Autodesk Fusion 360 part; units mm, degrees
note: some values were not read from the file. Set by a fixed rule: which sketch regions a step uses.
(part 3 of 8)
  spline S676 degree 3 poles (21.5017, -36.3646) (20.0626, -38.8974) (15.4509, -40.8816) (15.3621, -42.4125) knots 0 0 0 0 1 1 1 1
  spline S677 degree 3 poles (50.353, -26.1302) (50.6772, -26.1304) (51.0587, -26.408) (51.0577, -26.8365) knots 0 0 0 0 1 1 1 1
  spline S678 degree 3 poles (51.0577, -26.8365) (51.0567, -27.2899) (50.7639, -27.6151) (50.3584, -27.6166) knots 0 0 0 0 1 1 1 1
  spline S679 degree 3 poles (50.3584, -27.6166) (49.9248, -27.6184) (49.616, -27.2356) (49.6086, -26.8743) knots 0 0 0 0 1 1 1 1
  spline S680 degree 3 poles (49.6086, -26.8743) (49.5995, -26.4269) (49.9201, -26.13) (50.353, -26.1302) knots 0 0 0 0 1 1 1 1
  spline S681 degree 3 poles (51.5406, -53.5633) (51.8647, -53.5635) (52.2462, -53.8411) (52.2453, -54.2696) knots 0 0 0 0 1 1 1 1
  spline S682 degree 3 poles (52.2453, -54.2696) (52.2443, -54.723) (51.9515, -55.0482) (51.546, -55.0497) knots 0 0 0 0 1 1 1 1
  spline S683 degree 3 poles (51.546, -55.0497) (51.1123, -55.0515) (50.8035, -54.6687) (50.7962, -54.3074) knots 0 0 0 0 1 1 1 1
  spline S684 degree 3 poles (50.7962, -54.3074) (50.787, -53.86) (51.1077, -53.5631) (51.5406, -53.5633) knots 0 0 0 0 1 1 1 1
  spline S685 degree 3 poles (72.4312, -14.4997) (76.2469, -14.5855) (80.5372, -17.3952) (80.5274, -22.9562) knots 0 0 0 0 1 1 1 1
  spline S686 degree 3 poles (80.5274, -22.9562) (80.5194, -27.4888) (76.2962, -31.0017) (72.6195, -30.8225) knots 0 0 0 0 1 1 1 1
  spline S687 degree 3 poles (72.6195, -30.8225) (67.4693, -30.5715) (64.6367, -26.4712) (64.4292, -22.1695) knots 0 0 0 0 1 1 1 1
  spline S688 degree 3 poles (64.4292, -22.1695) (64.2167, -17.7617) (68.8119, -14.4186) (72.4312, -14.4997) knots 0 0 0 0 1 1 1 1
  spline S689 degree 3 poles (74.5023, -39.3772) (78.318, -39.4629) (82.6083, -42.2726) (82.5985, -47.8336) knots 0 0 0 0 1 1 1 1
  spline S690 degree 3 poles (82.5985, -47.8336) (82.5905, -52.3663) (78.3672, -55.8792) (74.6906, -55.7) knots 0 0 0 0 1 1 1 1
  spline S691 degree 3 poles (74.6906, -55.7) (69.5404, -55.449) (66.7077, -51.3486) (66.5003, -47.0469) knots 0 0 0 0 1 1 1 1
  spline S692 degree 3 poles (66.5003, -47.0469) (66.2878, -42.6392) (70.883, -39.2961) (74.5023, -39.3772) knots 0 0 0 0 1 1 1 1
  spline S693 degree 3 poles (73.2785, -58.2074) (82.3005, -57.5327) (89.9582, -48.2547) (90.1203, -35.5662) knots 0 0 0 0 1 1 1 1
  spline S694 degree 2 poles (90.1203, -35.5662) (87.4866, -35.4301) (84.6007, -35.3111) knots 0 0 0 1 1 1
  line L146 (84.6007, -35.3111) -> (84.471, -32.0483)
  spline S695 degree 2 poles (84.471, -32.0483) (87.0415, -31.8252) (89.6592, -31.806) knots 0 0 0 1 1 1
  spline S696 degree 3 poles (89.6592, -31.806) (89.4171, -23.0769) (80.9156, -11.9731) (70.8766, -11.9613) knots 0 0 0 0 1 1 1 1
  spline S697 degree 3 poles (70.8766, -11.9613) (65.914, -11.9571) (60.8467, -16.8048) (60.6556, -22.2308) knots 0 0 0 0 1 1 1 1
  spline S698 degree 3 poles (60.6556, -22.2308) (60.4942, -26.8139) (64.4737, -30.3857) (65.4815, -34.4267) knots 0 0 0 0 1 1 1 1
  spline S699 degree 2 poles (65.4815, -34.4267) (66.1184, -34.46) (67.0382, -34.426) knots 0 0 0 1 1 1
  line L147 (67.0382, -34.426) -> (67.0737, -37.0293)
  spline S700 degree 2 poles (67.0737, -37.0293) (65.9901, -37.0984) (65.537, -37.0984) knots 0 0 0 1 1 1
  spline S701 degree 3 poles (65.537, -37.0984) (65.3316, -41.8108) (62.9469, -42.7703) (63.0893, -47.5705) knots 0 0 0 0 1 1 1 1
  spline S702 degree 3 poles (63.0893, -47.5705) (63.3075, -54.9251) (68.8259, -58.3029) (73.2785, -58.2074) knots 0 0 0 0 1 1 1 1
  spline S703 degree 3 poles (75.2555, -32.5471) (76.3242, -32.5305) (77.1113, -32.4934) (78.4498, -32.4976) knots 0 0 0 0 1 1 1 1
  spline S704 degree 3 poles (78.4498, -32.4976) (79.3002, -32.4997) (79.9929, -33.259) (80.0372, -34.5532) knots 0 0 0 0 1 1 1 1
  spline S705 degree 3 poles (80.0372, -34.5532) (80.0711, -35.5384) (79.5067, -36.6633) (78.5769, -36.7117) knots 0 0 0 0 1 1 1 1
  spline S706 degree 3 poles (78.5769, -36.7117) (77.3189, -36.7771) (76.4003, -36.7367) (74.9094, -36.745) knots 0 0 0 0 1 1 1 1
  spline S707 degree 3 poles (74.9094, -36.745) (73.8775, -36.7492) (73.3711, -35.5379) (73.3735, -34.5911) knots 0 0 0 0 1 1 1 1
  spline S708 degree 3 poles (73.3735, -34.5911) (73.3763, -33.5178) (73.9925, -32.5674) (75.2555, -32.549) knots 0 0 0 0 1 1 1 1
  line L148 (75.2555, -32.549) -> (75.2555, -32.5471)
  spline S709 degree 3 poles (23.3685, -73.0015) (22.2201, -71.8744) (21.4826, -70.2942) (21.3371, -68.6485) knots 0 0 0 0 1 1 1 1
  spline S710 degree 3 poles (21.3371, -68.6485) (21.2174, -67.2961) (21.5085, -65.8738) (22.2993, -64.8005) knots 0 0 0 0 1 1 1 1
  spline S711 degree 3 poles (22.2993, -64.8005) (22.6948, -64.2639) (23.2101, -63.822) (23.7995, -63.5458) knots 0 0 0 0 1 1 1 1
  spline S712 degree 3 poles (23.7995, -63.5458) (24.3889, -63.2696) (25.0523, -63.1624) (25.6902, -63.2644) knots 0 0 0 0 1 1 1 1
  spline S713 degree 3 poles (25.6902, -63.2644) (25.9412, -63.3046) (26.1875, -63.3765) (26.4223, -63.4781) knots 0 0 0 0 1 1 1 1
  line L149 (26.4223, -63.4781) -> (26.3432, -66.5101)
  spline S714 degree 3 poles (26.3432, -66.5101) (26.3414, -66.5806) (26.3399, -66.6516) (26.3518, -66.721) knots 0 0 0 0 1 1 1 1
  spline S715 degree 3 poles (26.3518, -66.721) (26.3636, -66.7904) (26.3893, -66.8584) (26.4339, -66.9111) knots 0 0 0 0 1 1 1 1
  spline S716 degree 3 poles (26.4339, -66.9111) (26.4838, -66.97) (26.5544, -67.0063) (26.6274, -67.0245) knots 0 0 0 0 1 1 1 1
  spline S717 degree 3 poles (26.6274, -67.0245) (26.7003, -67.0427) (26.7761, -67.044) (26.851, -67.0447) knots 0 0 0 0 1 1 1 1
  line L150 (26.851, -67.0447) -> (30.6238, -67.0829)
  spline S718 degree 3 poles (30.6238, -67.0829) (30.7378, -67.084) (30.852, -67.0875) (30.9657, -67.078) knots 0 0 0 0 1 1 1 1
  spline S719 degree 3 poles (30.9657, -67.078) (31.0793, -67.0685) (31.1951, -67.0436) (31.2905, -66.9778) knots 0 0 0 0 1 1 1 1
  spline S720 degree 3 poles (31.2905, -66.9778) (31.3594, -66.9303) (31.4152, -66.8619) (31.4495, -66.7831) knots 0 0 0 0 1 1 1 1
  spline S721 degree 3 poles (31.4495, -66.7831) (31.4838, -66.7042) (31.4964, -66.615) (31.4855, -66.5291) knots 0 0 0 0 1 1 1 1
  line L151 (31.4855, -66.5291) -> (31.5307, -64.1427)
  spline S722 degree 3 poles (31.5307, -64.1427) (31.5118, -64.0654) (31.5145, -63.9824) (31.5385, -63.9067) knots 0 0 0 0 1 1 1 1
  spline S723 degree 3 poles (31.5385, -63.9067) (31.5625, -63.8309) (31.6077, -63.7628) (31.6669, -63.7129) knots 0 0 0 0 1 1 1 1
  spline S724 degree 3 poles (31.6669, -63.7129) (31.7303, -63.6596) (31.8081, -63.6279) (31.8876, -63.6109) knots 0 0 0 0 1 1 1 1
  spline S725 degree 3 poles (31.8876, -63.6109) (31.9671, -63.5939) (32.0486, -63.5911) (32.1296, -63.5886) knots 0 0 0 0 1 1 1 1
  line L152 (32.1296, -63.5886) -> (36.4643, -63.4554)
  spline S726 degree 3 poles (36.4643, -63.4554) (36.4791, -62.6007) (36.898, -61.7642) (37.5596, -61.2684) knots 0 0 0 0 1 1 1 1
  spline S727 degree 3 poles (37.5596, -61.2684) (37.8482, -61.052) (38.1798, -60.9005) (38.5261, -60.8212) knots 0 0 0 0 1 1 1 1
  spline S728 degree 3 poles (38.5261, -60.8212) (38.8723, -60.7419) (39.2297, -60.7387) (39.584, -60.7443) knots 0 0 0 0 1 1 1 1
  line L153 (39.584, -60.7443) -> (51.3262, -60.9286)
  spline S729 degree 3 poles (51.3262, -60.9286) (51.8918, -60.9406) (52.451, -61.1692) (52.8762, -61.562) knots 0 0 0 0 1 1 1 1
  spline S730 degree 3 poles (52.8762, -61.562) (53.2339, -61.8924) (53.4915, -62.3265) (53.7043, -62.7746) knots 0 0 0 0 1 1 1 1
  spline S731 degree 3 poles (53.7043, -62.7746) (53.8166, -63.011) (53.9182, -63.2535) (54.0434, -63.4826) knots 0 0 0 0 1 1 1 1
  spline S732 degree 3 poles (54.0434, -63.4826) (54.1686, -63.7117) (54.3195, -63.9292) (54.5148, -64.0953) knots 0 0 0 0 1 1 1 1
  spline S733 degree 3 poles (54.5148, -64.0953) (54.8537, -64.3832) (55.2965, -64.4935) (55.727, -64.5627) knots 0 0 0 0 1 1 1 1
  spline S734 degree 3 poles (55.727, -64.5627) (56.3986, -64.6707) (57.0794, -64.6956) (57.7585, -64.7155) knots 0 0 0 0 1 1 1 1
  line L154 (57.7585, -64.7155) -> (115.2201, -66.3956)
  spline S735 degree 3 poles (115.2201, -66.3956) (115.6074, -66.4069) (115.9977, -66.4549) (116.381, -66.3956) knots 0 0 0 0 1 1 1 1
  spline S736 degree 3 poles (116.381, -66.3956) (116.6412, -66.3553) (116.8939, -66.2531) (117.1065, -66.0901) knots 0 0 0 0 1 1 1 1
  spline S737 degree 3 poles (117.1065, -66.0901) (117.5006, -65.7881) (117.7284, -65.3094) (117.9771, -64.8682) knots 0 0 0 0 1 1 1 1
  spline S738 degree 3 poles (117.9771, -64.8682) (118.2594, -64.3676) (118.5967, -63.8834) (119.0603, -63.5661) knots 0 0 0 0 1 1 1 1
  spline S739 degree 3 poles (119.0603, -63.5661) (119.4759, -63.2816) (119.982, -63.1465) (120.4761, -63.1881) knots 0 0 0 0 1 1 1 1
  line L155 (120.4761, -63.1881) -> (132.583, -63.5028)
  spline S740 degree 3 poles (132.583, -63.5028) (133.2403, -63.4478) (133.9156, -63.7151) (134.3755, -64.2125) knots 0 0 0 0 1 1 1 1
  spline S741 degree 3 poles (134.3755, -64.2125) (134.8733, -64.7509) (135.1048, -65.5483) (134.9778, -66.2876) knots 0 0 0 0 1 1 1 1
  line L156 (134.9778, -66.2876) -> (139.3853, -66.5036)
  spline S742 degree 3 poles (139.3853, -66.5036) (139.5114, -66.5097) (139.6383, -66.5162) (139.7611, -66.5467) knots 0 0 0 0 1 1 1 1
  spline S743 degree 3 poles (139.7611, -66.5467) (139.8839, -66.5773) (140.0037, -66.6337) (140.0932, -66.7273) knots 0 0 0 0 1 1 1 1
  spline S744 degree 3 poles (140.0932, -66.7273) (140.1909, -66.8294) (140.2466, -66.9694) (140.2731, -67.1117) knots 0 0 0 0 1 1 1 1
  spline S745 degree 3 poles (140.2731, -67.1117) (140.2995, -67.2539) (140.299, -67.4) (140.2984, -67.545) knots 0 0 0 0 1 1 1 1
  line L157 (140.2984, -67.545) -> (140.2899, -69.7019)
  spline S746 degree 3 poles (140.2899, -69.7019) (140.2895, -69.8149) (140.2888, -69.9287) (140.3062, -70.0402) knots 0 0 0 0 1 1 1 1
  spline S747 degree 3 poles (140.3062, -70.0402) (140.3237, -70.1518) (140.3608, -70.2625) (140.4299, -70.3491) knots 0 0 0 0 1 1 1 1
  spline S748 degree 3 poles (140.4299, -70.3491) (140.4775, -70.4086) (140.5395, -70.4552) (140.6085, -70.4833) knots 0 0 0 0 1 1 1 1
  spline S749 degree 3 poles (140.6085, -70.4833) (140.6774, -70.5113) (140.7531, -70.5207) (140.8264, -70.5103) knots 0 0 0 0 1 1 1 1
  line L158 (140.8264, -70.5103) -> (144.5244, -70.5643)
  spline S750 degree 3 poles (144.5244, -70.5643) (144.685, -70.5887) (144.8549, -70.5347) (144.9758, -70.4208) knots 0 0 0 0 1 1 1 1
  spline S751 degree 3 poles (144.9758, -70.4208) (145.114, -70.2906) (145.1837, -70.0845) (145.1546, -69.8917) knots 0 0 0 0 1 1 1 1
  line L159 (145.1546, -69.8917) -> (145.2484, -67.1238)
  spline S752 degree 3 poles (145.2484, -67.1238) (145.4352, -66.9982) (145.6371, -66.8973) (145.8476, -66.8242) knots 0 0 0 0 1 1 1 1
  spline S753 degree 3 poles (145.8476, -66.8242) (146.4322, -66.6212) (147.0785, -66.639) (147.6628, -66.8426) knots 0 0 0 0 1 1 1 1
  spline S754 degree 3 poles (147.6628, -66.8426) (148.2471, -67.0463) (148.769, -67.4308) (149.1755, -67.9173) knots 0 0 0 0 1 1 1 1
  spline S755 degree 3 poles (149.1755, -67.9173) (149.9885, -68.8903) (150.3196, -70.2311) (150.3052, -71.5268) knots 0 0 0 0 1 1 1 1
  spline S756 degree 3 poles (150.3052, -71.5268) (150.2851, -73.328) (149.627, -75.1136) (148.4877, -76.4578) knots 0 0 0 0 1 1 1 1
  line L160 (148.4877, -76.4578) -> (134.4681, -76.4409)
  spline S757 degree 3 poles (134.4681, -76.4409) (134.3422, -76.9072) (134.0363, -77.3167) (133.6355, -77.5556) knots 0 0 0 0 1 1 1 1
  spline S758 degree 3 poles (133.6355, -77.5556) (133.3442, -77.7292) (133.0111, -77.813) (132.6779, -77.848) knots 0 0 0 0 1 1 1 1
  spline S759 degree 3 poles (132.6779, -77.848) (132.3448, -77.8829) (132.009, -77.8712) (131.6744, -77.8603) knots 0 0 0 0 1 1 1 1
  line L161 (131.6744, -77.8603) -> (116.3387, -77.3573)
  spline S760 degree 3 poles (116.3387, -77.3573) (116.1319, -77.3505) (115.9238, -77.3446) (115.7192, -77.3771) knots 0 0 0 0 1 1 1 1
  spline S761 degree 3 poles (115.7192, -77.3771) (115.5146, -77.4095) (115.3125, -77.4818) (115.1471, -77.6126) knots 0 0 0 0 1 1 1 1
  spline S762 degree 3 poles (115.1471, -77.6126) (115.0025, -77.727) (114.8892, -77.8848) (114.8241, -78.0624) knots 0 0 0 0 1 1 1 1
  spline S763 degree 3 poles (114.8241, -78.0624) (114.7589, -78.24) (114.7422, -78.437) (114.7763, -78.624) knots 0 0 0 0 1 1 1 1
  line L162 (114.7763, -78.624) -> (114.7162, -87.671)
  spline S764 degree 3 poles (114.7162, -87.671) (114.6628, -88.1799) (114.8565, -88.7106) (115.2197, -89.0511) knots 0 0 0 0 1 1 1 1
  spline S765 degree 3 poles (115.2197, -89.0511) (115.4965, -89.3106) (115.8654, -89.4587) (116.2362, -89.4591) knots 0 0 0 0 1 1 1 1
  line L163 (116.2362, -89.4591) -> (132.4279, -90.0963)
  spline S766 degree 3 poles (132.4279, -90.0963) (132.8986, -90.0815) (133.3726, -90.2466) (133.7419, -90.5541) knots 0 0 0 0 1 1 1 1
  spline S767 degree 3 poles (133.7419, -90.5541) (134.1545, -90.8976) (134.4311, -91.4166) (134.4945, -91.9662) knots 0 0 0 0 1 1 1 1
  line L164 (134.4945, -91.9662) -> (148.1256, -92.4599)
  spline S768 degree 3 poles (148.1256, -92.4599) (148.8324, -93.2896) (149.3295, -94.3154) (149.5527, -95.4047) knots 0 0 0 0 1 1 1 1
  spline S769 degree 3 poles (149.5527, -95.4047) (149.7758, -96.4941) (149.7244, -97.6444) (149.4052, -98.7069) knots 0 0 0 0 1 1 1 1
  spline S770 degree 3 poles (149.4052, -98.7069) (149.0854, -99.7712) (148.4747, -100.7686) (147.5774, -101.3635) knots 0 0 0 0 1 1 1 1
  spline S771 degree 3 poles (147.5774, -101.3635) (146.721, -101.9313) (145.6312, -102.0927) (144.6592, -101.7955) knots 0 0 0 0 1 1 1 1
  line L165 (144.6592, -101.7955) -> (144.5317, -98.7315)
  spline S772 degree 3 poles (144.5317, -98.7315) (144.494, -98.5283) (144.3864, -98.3402) (144.2334, -98.21) knots 0 0 0 0 1 1 1 1
  spline S773 degree 3 poles (144.2334, -98.21) (144.0917, -98.0894) (143.9121, -98.0189) (143.73, -98.0125) knots 0 0 0 0 1 1 1 1
  line L166 (143.73, -98.0125) -> (139.8707, -98.0758)
  spline S774 degree 3 poles (139.8707, -98.0758) (139.7838, -98.054) (139.6903, -98.0623) (139.6081, -98.099) knots 0 0 0 0 1 1 1 1
  spline S775 degree 3 poles (139.6081, -98.099) (139.5259, -98.1358) (139.4553, -98.2008) (139.4098, -98.2817) knots 0 0 0 0 1 1 1 1
  spline S776 degree 3 poles (139.4098, -98.2817) (139.3572, -98.3752) (139.3389, -98.4893) (139.3592, -98.5957) knots 0 0 0 0 1 1 1 1
  line L167 (139.3592, -98.5957) -> (139.3379, -101.0866)
  spline S777 degree 3 poles (139.3379, -101.0866) (139.337, -101.196) (139.3371, -101.306) (139.3207, -101.414) knots 0 0 0 0 1 1 1 1
  spline S778 degree 3 poles (139.3207, -101.414) (139.3042, -101.522) (139.2689, -101.6303) (139.199, -101.7111) knots 0 0 0 0 1 1 1 1
  spline S779 degree 3 poles (139.199, -101.7111) (139.1442, -101.7743) (139.0692, -101.8179) (138.9892, -101.833) knots 0 0 0 0 1 1 1 1
  spline S780 degree 3 poles (138.9892, -101.833) (138.9092, -101.8482) (138.8245, -101.8348) (138.7523, -101.7955) knots 0 0 0 0 1 1 1 1
  line L168 (138.7523, -101.7955) -> (134.2379, -101.7601)
  spline S781 degree 3 poles (134.2379, -101.7601) (134.2725, -102.4664) (133.9962, -103.1829) (133.5036, -103.6639) knots 0 0 0 0 1 1 1 1
  spline S782 degree 3 poles (133.5036, -103.6639) (132.998, -104.1575) (132.2742, -104.3924) (131.5923, -104.2841) knots 0 0 0 0 1 1 1 1
  line L169 (131.5923, -104.2841) -> (119.2583, -103.9786)
  spline S783 degree 3 poles (119.2583, -103.9786) (118.7444, -103.8806) (118.2487, -103.6772) (117.8073, -103.3832) knots 0 0 0 0 1 1 1 1
  spline S784 degree 3 poles (117.8073, -103.3832) (116.7983, -102.7111) (116.0967, -101.5504) (115.9458, -100.3036) knots 0 0 0 0 1 1 1 1
  line L170 (115.9458, -100.3036) -> (56.2679, -98.6327)
  spline S785 degree 3 poles (56.2679, -98.6327) (55.8319, -98.6205) (55.3941, -98.5951) (54.9602, -98.6429) knots 0 0 0 0 1 1 1 1
  spline S786 degree 3 poles (54.9602, -98.6429) (54.6434, -98.6777) (54.328, -98.7575) (54.0452, -98.9117) knots 0 0 0 0 1 1 1 1
  spline S787 degree 3 poles (54.0452, -98.9117) (53.7463, -99.0747) (53.4855, -99.3242) (53.3294, -99.6382) knots 0 0 0 0 1 1 1 1
  spline S788 degree 3 poles (53.3294, -99.6382) (53.1481, -100.0025) (53.1141, -100.4327) (52.9316, -100.7963) knots 0 0 0 0 1 1 1 1
  spline S789 degree 3 poles (52.9316, -100.7963) (52.8073, -101.0437) (52.6153, -101.2529) (52.3847, -101.3923) knots 0 0 0 0 1 1 1 1
  spline S790 degree 3 poles (52.3847, -101.3923) (52.1541, -101.5316) (51.8857, -101.6006) (51.62, -101.5888) knots 0 0 0 0 1 1 1 1
  line L171 (51.62, -101.5888) -> (38.2822, -101.4082)
  spline S791 degree 3 poles (38.2822, -101.4082) (38.1033, -101.4058) (37.9235, -101.3983) (37.7488, -101.358) knots 0 0 0 0 1 1 1 1
  spline S792 degree 3 poles (37.7488, -101.358) (37.5741, -101.3177) (37.4064, -101.2475) (37.2488, -101.1583) knots 0 0 0 0 1 1 1 1
  spline S793 degree 3 poles (37.2488, -101.1583) (36.8107, -100.9104) (36.4463, -100.5206) (36.2178, -100.0555) knots 0 0 0 0 1 1 1 1
  spline S794 degree 3 poles (36.2178, -100.0555) (35.9894, -99.5904) (35.8979, -99.052) (35.959, -98.5324) knots 0 0 0 0 1 1 1 1
  line L172 (35.959, -98.5324) -> (31.6131, -98.6049)
  spline S795 degree 3 poles (31.6131, -98.6049) (31.5119, -98.6066) (31.4103, -98.6079) (31.3101, -98.5929) knots 0 0 0 0 1 1 1 1
  spline S796 degree 3 poles (31.3101, -98.5929) (31.2099, -98.5779) (31.1108, -98.5463) (31.0254, -98.4892) knots 0 0 0 0 1 1 1 1
  spline S797 degree 3 poles (31.0254, -98.4892) (30.9406, -98.4325) (30.8709, -98.3512) (30.826, -98.2566) knots 0 0 0 0 1 1 1 1
  spline S798 degree 3 poles (30.826, -98.2566) (30.7811, -98.1621) (30.7611, -98.0546) (30.7689, -97.9492) knots 0 0 0 0 1 1 1 1
  line L173 (30.7689, -97.9492) -> (30.5725, -95.1552)
  spline S799 degree 3 poles (30.5725, -95.1552) (30.5791, -94.9521) (30.5069, -94.7475) (30.3761, -94.5982) knots 0 0 0 0 1 1 1 1
  spline S800 degree 3 poles (30.3761, -94.5982) (30.2413, -94.4444) (30.0457, -94.3515) (29.847, -94.3467) knots 0 0 0 0 1 1 1 1
  line L174 (29.847, -94.3467) -> (26.5432, -94.3467)
  spline S801 degree 3 poles (26.5432, -94.3467) (26.3535, -94.3319) (26.1591, -94.414) (26.0317, -94.5627) knots 0 0 0 0 1 1 1 1
  spline S802 degree 3 poles (26.0317, -94.5627) (25.9082, -94.707) (25.8501, -94.9108) (25.8778, -95.1027) knots 0 0 0 0 1 1 1 1
  line L175 (25.8778, -95.1027) -> (25.9042, -98.2099)
  spline S803 degree 3 poles (25.9042, -98.2099) (25.7162, -98.2716) (25.5234, -98.3171) (25.3283, -98.3457) knots 0 0 0 0 1 1 1 1
  spline S804 degree 3 poles (25.3283, -98.3457) (24.1437, -98.5197) (22.9086, -98.0401) (22.0479, -97.1659) knots 0 0 0 0 1 1 1 1
  spline S805 degree 3 poles (22.0479, -97.1659) (21.1872, -96.2916) (20.694, -95.0535) (20.6085, -93.7977) knots 0 0 0 0 1 1 1 1
  spline S806 degree 3 poles (20.6085, -93.7977) (20.5409, -92.8051) (20.7186, -91.795) (21.1194, -90.8936) knots 0 0 0 0 1 1 1 1
  spline S807 degree 3 poles (21.1194, -90.8936) (21.5202, -89.9923) (22.1432, -89.2016) (22.9106, -88.6204) knots 0 0 0 0 1 1 1 1
  line L176 (22.9106, -88.6204) -> (36.0543, -88.6414)
  spline S808 degree 3 poles (36.0543, -88.6414) (36.2423, -88.3197) (36.4933, -88.039) (36.7871, -87.8221) knots 0 0 0 0 1 1 1 1
  spline S809 degree 3 poles (36.7871, -87.8221) (37.3131, -87.4338) (37.9769, -87.2578) (38.6149, -87.3376) knots 0 0 0 0 1 1 1 1
  line L177 (38.6149, -87.3376) -> (54.2246, -87.6077)
  spline S810 degree 3 poles (54.2246, -87.6077) (54.4295, -87.6112) (54.6346, -87.618) (54.8393, -87.6072) knots 0 0 0 0 1 1 1 1
  spline S811 degree 3 poles (54.8393, -87.6072) (55.044, -87.5964) (55.2513, -87.5652) (55.4368, -87.4734) knots 0 0 0 0 1 1 1 1
  spline S812 degree 3 poles (55.4368, -87.4734) (55.6027, -87.3914) (55.7466, -87.2608) (55.8483, -87.1003) knots 0 0 0 0 1 1 1 1
  spline S813 degree 3 poles (55.8483, -87.1003) (55.9499, -86.9398) (56.009, -86.7497) (56.0172, -86.557) knots 0 0 0 0 1 1 1 1
  line L178 (56.0172, -86.557) -> (56.1022, -76.9699)
  spline S814 degree 3 poles (56.1022, -76.9699) (56.1428, -76.6491) (56.0582, -76.3127) (55.8721, -76.0551) knots 0 0 0 0 1 1 1 1
  spline S815 degree 3 poles (55.8721, -76.0551) (55.7532, -75.8904) (55.5945, -75.7579) (55.4151, -75.6734) knots 0 0 0 0 1 1 1 1
  spline S816 degree 3 poles (55.4151, -75.6734) (55.2358, -75.589) (55.0361, -75.5527) (54.8403, -75.5691) knots 0 0 0 0 1 1 1 1
  line L179 (54.8403, -75.5691) -> (39.2114, -75.1109)
  spline S817 degree 3 poles (39.2114, -75.1109) (38.6875, -75.1125) (38.1643, -74.941) (37.7339, -74.6265) knots 0 0 0 0 1 1 1 1
  spline S818 degree 3 poles (37.7339, -74.6265) (37.2427, -74.2675) (36.8765, -73.7231) (36.7182, -73.1161) knots 0 0 0 0 1 1 1 1
  line L180 (36.7182, -73.1161) -> (23.3685, -73.0015)
  spline S819 degree 3 poles (61.6296, -85.4421) (62.5295, -85.7248) (63.5344, -85.6159) (64.3607, -85.1461) knots 0 0 0 0 1 1 1 1
  spline S820 degree 3 poles (64.3607, -85.1461) (65.1869, -84.6762) (65.8243, -83.8512) (66.0929, -82.904) knots 0 0 0 0 1 1 1 1
  spline S821 degree 3 poles (66.0929, -82.904) (66.3616, -81.9568) (66.2581, -80.899) (65.8117, -80.0293) knots 0 0 0 0 1 1 1 1
  spline S822 degree 3 poles (65.8117, -80.0293) (65.3653, -79.1596) (64.5816, -78.4887) (63.6817, -78.2059) knots 0 0 0 0 1 1 1 1
  spline S823 degree 3 poles (63.6817, -78.2059) (62.7818, -77.9232) (61.7769, -78.0321) (60.9507, -78.5019) knots 0 0 0 0 1 1 1 1
  spline S824 degree 3 poles (60.9507, -78.5019) (60.1244, -78.9718) (59.487, -79.7968) (59.2184, -80.744) knots 0 0 0 0 1 1 1 1
  spline S825 degree 3 poles (59.2184, -80.744) (58.9498, -81.6912) (59.0533, -82.749) (59.4996, -83.6187) knots 0 0 0 0 1 1 1 1
  spline S826 degree 3 poles (59.4996, -83.6187) (59.946, -84.4884) (60.7297, -85.1593) (61.6296, -85.4421) knots 0 0 0 0 1 1 1 1
  spline S827 degree 3 poles (107.0839, -86.9677) (107.9838, -87.2504) (108.9887, -87.1415) (109.815, -86.6716) knots 0 0 0 0 1 1 1 1
  spline S828 degree 3 poles (109.815, -86.6716) (110.6412, -86.2018) (111.2786, -85.3768) (111.5472, -84.4296) knots 0 0 0 0 1 1 1 1
  spline S829 degree 3 poles (111.5472, -84.4296) (111.8159, -83.4824) (111.7124, -82.4246) (111.266, -81.5549) knots 0 0 0 0 1 1 1 1
  spline S830 degree 3 poles (111.266, -81.5549) (110.8196, -80.6852) (110.0359, -80.0142) (109.136, -79.7315) knots 0 0 0 0 1 1 1 1
  spline S831 degree 3 poles (109.136, -79.7315) (108.2362, -79.4487) (107.2312, -79.5577) (106.405, -80.0275) knots 0 0 0 0 1 1 1 1
  spline S832 degree 3 poles (106.405, -80.0275) (105.5787, -80.4973) (104.9413, -81.3223) (104.6727, -82.2695) knots 0 0 0 0 1 1 1 1
  spline S833 degree 3 poles (104.6727, -82.2695) (104.4041, -83.2168) (104.5076, -84.2745) (104.9539, -85.1443) knots 0 0 0 0 1 1 1 1
  spline S834 degree 3 poles (104.9539, -85.1443) (105.4003, -86.014) (106.1841, -86.6849) (107.0839, -86.9677) knots 0 0 0 0 1 1 1 1
  spline S835 degree 3 poles (70.4371, -72.9822) (70.1477, -72.9883) (69.8625, -73.1192) (69.6613, -73.3381) knots 0 0 0 0 1 1 1 1
  spline S836 degree 3 poles (69.6613, -73.3381) (69.46, -73.557) (69.3451, -73.8613) (69.3488, -74.1659) knots 0 0 0 0 1 1 1 1
  spline S837 degree 3 poles (69.3488, -74.1659) (69.3517, -74.4139) (69.4321, -74.6603) (69.5745, -74.8579) knots 0 0 0 0 1 1 1 1
  spline S838 degree 3 poles (69.5745, -74.8579) (69.717, -75.0556) (69.9207, -75.2034) (70.1468, -75.2732) knots 0 0 0 0 1 1 1 1
  line L181 (70.1468, -75.2732) -> (100.9091, -75.9224)
  spline S839 degree 3 poles (100.9091, -75.9224) (101.1096, -75.8838) (101.2987, -75.7822) (101.4459, -75.634) knots 0 0 0 0 1 1 1 1
  spline S840 degree 3 poles (101.4459, -75.634) (101.5931, -75.4857) (101.698, -75.2914) (101.7435, -75.0823) knots 0 0 0 0 1 1 1 1
  spline S841 degree 3 poles (101.7435, -75.0823) (101.8202, -74.73) (101.7196, -74.3405) (101.4841, -74.0775) knots 0 0 0 0 1 1 1 1
  spline S842 degree 3 poles (101.4841, -74.0775) (101.2485, -73.8145) (100.885, -73.686) (100.5464, -73.7459) knots 0 0 0 0 1 1 1 1
  line L182 (100.5464, -73.7459) -> (99.6395, -73.7077)
  line L183 (99.6395, -73.7077) -> (99.6757, -74.1277)
  line L184 (99.6757, -74.1277) -> (97.6806, -74.1277)
  line L185 (97.6806, -74.1277) -> (97.6806, -73.6695)
  line L186 (97.6806, -73.6695) -> (96.0118, -73.6313)
  line L187 (96.0118, -73.6313) -> (96.0118, -74.0895)
  line L188 (96.0118, -74.0895) -> (93.8715, -74.0895)
  line L189 (93.8715, -74.0895) -> (93.8353, -73.5549)
  line L190 (93.8353, -73.5549) -> (92.2391, -73.5549)
  line L191 (92.2391, -73.5549) -> (92.2391, -74.0513)
  line L192 (92.2391, -74.0513) -> (90.1351, -73.9749)
  line L193 (90.1351, -73.9749) -> (90.1714, -73.4785)
  line L194 (90.1714, -73.4785) -> (88.6115, -73.4022)
  line L195 (88.6115, -73.4022) -> (88.6115, -73.8604)
  line L196 (88.6115, -73.8604) -> (86.5437, -73.784)
  line L197 (86.5437, -73.784) -> (86.5437, -73.364)
  line L198 (86.5437, -73.364) -> (84.8025, -73.364)
  line L199 (84.8025, -73.364) -> (84.8387, -73.7459)
  line L200 (84.8387, -73.7459) -> (82.6984, -73.6313)
  line L201 (82.6984, -73.6313) -> (82.6984, -73.1731)
  line L202 (82.6984, -73.1731) -> (81.0297, -73.1349)
  line L203 (81.0297, -73.1349) -> (81.0297, -73.6313)
  line L204 (81.0297, -73.6313) -> (78.9983, -73.5931)
  line L205 (78.9983, -73.5931) -> (79.0345, -73.1349)
  line L206 (79.0345, -73.1349) -> (77.1119, -73.1349)
  line L207 (77.1119, -73.1349) -> (77.1482, -73.5549)
  line L208 (77.1482, -73.5549) -> (75.1892, -73.4786)
  line L209 (75.1892, -73.4786) -> (75.1892, -73.0203)
  line L210 (75.1892, -73.0203) -> (73.3754, -72.9822)
  line L211 (73.3754, -72.9822) -> (73.3754, -73.4404)
  line L212 (73.3754, -73.4404) -> (71.4528, -73.4022)
  line L213 (71.4528, -73.4022) -> (71.4891, -72.9822)
  line L214 (71.4891, -72.9822) -> (70.4371, -72.9822)
  spline S843 degree 3 poles (70.2066, -88.9065) (69.9173, -88.9126) (69.6321, -89.0435) (69.4308, -89.2624) knots 0 0 0 0 1 1 1 1
  spline S844 degree 3 poles (69.4308, -89.2624) (69.2296, -89.4813) (69.1147, -89.7856) (69.1183, -90.0902) knots 0 0 0 0 1 1 1 1
  spline S845 degree 3 poles (69.1183, -90.0902) (69.1213, -90.3383) (69.2016, -90.5846) (69.3441, -90.7823) knots 0 0 0 0 1 1 1 1
  spline S846 degree 3 poles (69.3441, -90.7823) (69.4865, -90.9799) (69.6902, -91.1277) (69.9164, -91.1976) knots 0 0 0 0 1 1 1 1
  line L215 (69.9164, -91.1976) -> (100.6787, -91.8467)
  spline S847 degree 3 poles (100.6787, -91.8467) (100.8791, -91.8081) (101.0682, -91.7065) (101.2154, -91.5583) knots 0 0 0 0 1 1 1 1
  spline S848 degree 3 poles (101.2154, -91.5583) (101.3627, -91.41) (101.4675, -91.2157) (101.513, -91.0066) knots 0 0 0 0 1 1 1 1
  spline S849 degree 3 poles (101.513, -91.0066) (101.5897, -90.6544) (101.4892, -90.2648) (101.2536, -90.0018) knots 0 0 0 0 1 1 1 1
  spline S850 degree 3 poles (101.2536, -90.0018) (101.0181, -89.7389) (100.6545, -89.6103) (100.3159, -89.6702) knots 0 0 0 0 1 1 1 1
  line L216 (100.3159, -89.6702) -> (99.409, -89.632)
  line L217 (99.409, -89.632) -> (99.4453, -90.052)
  line L218 (99.4453, -90.052) -> (97.4501, -90.052)
  line L219 (97.4501, -90.052) -> (97.4501, -89.5938)
  line L220 (97.4501, -89.5938) -> (95.7814, -89.5556)
  line L221 (95.7814, -89.5556) -> (95.7814, -90.0138)
  line L222 (95.7814, -90.0138) -> (93.6411, -90.0138)
  line L223 (93.6411, -90.0138) -> (93.6048, -89.4792)
  line L224 (93.6048, -89.4792) -> (92.0087, -89.4792)
  line L225 (92.0087, -89.4792) -> (92.0087, -89.9756)
  line L226 (92.0087, -89.9756) -> (89.9046, -89.8993)
  line L227 (89.9046, -89.8993) -> (89.9409, -89.4029)
  line L228 (89.9409, -89.4029) -> (88.381, -89.3265)
  line L229 (88.381, -89.3265) -> (88.381, -89.7847)
  line L230 (88.381, -89.7847) -> (86.3133, -89.7084)
  line L231 (86.3133, -89.7084) -> (86.3133, -89.2883)
  line L232 (86.3133, -89.2883) -> (84.572, -89.2883)
  line L233 (84.572, -89.2883) -> (84.6083, -89.6702)
  line L234 (84.6083, -89.6702) -> (82.468, -89.5556)
  line L235 (82.468, -89.5556) -> (82.468, -89.0974)
  line L236 (82.468, -89.0974) -> (80.7993, -89.0592)
  line L237 (80.7993, -89.0592) -> (80.7993, -89.5556)
  line L238 (80.7993, -89.5556) -> (78.7678, -89.5174)
  line L239 (78.7678, -89.5174) -> (78.8041, -89.0592)
  line L240 (78.8041, -89.0592) -> (76.8814, -89.0592)
  line L241 (76.8814, -89.0592) -> (76.9177, -89.4792)
  line L242 (76.9177, -89.4792) -> (74.9588, -89.4029)
  line L243 (74.9588, -89.4029) -> (74.9588, -88.9447)
  line L244 (74.9588, -88.9447) -> (73.145, -88.9065)
  line L245 (73.145, -88.9065) -> (73.145, -89.3647)
  line L246 (73.145, -89.3647) -> (71.2223, -89.3265)
  line L247 (71.2223, -89.3265) -> (71.2586, -88.9065)
  line L248 (71.2586, -88.9065) -> (70.2066, -88.9065)
  spline S851 degree 3 poles (40.0515, -65.8778) (39.9072, -65.8671) (39.7599, -65.9107) (39.6421, -65.9989) knots 0 0 0 0 1 1 1 1
  spline S852 degree 3 poles (39.6421, -65.9989) (39.5107, -66.0973) (39.4176, -66.2509) (39.3882, -66.4178) knots 0 0 0 0 1 1 1 1
  line L249 (39.3882, -66.4178) -> (39.3644, -69.1877)
  spline S853 degree 3 poles (39.3644, -69.1877) (39.3568, -69.3937) (39.43, -69.6017) (39.5633, -69.7528) knots 0 0 0 0 1 1 1 1
  spline S854 degree 3 poles (39.5633, -69.7528) (39.7182, -69.9283) (39.9524, -70.0225) (40.179, -70.0004) knots 0 0 0 0 1 1 1 1
  line L250 (40.179, -70.0004) -> (49.3108, -69.9688)
  spline S855 degree 3 poles (49.3108, -69.9688) (49.7498, -69.8504) (50.1478, -69.5705) (50.4197, -69.1889) knots 0 0 0 0 1 1 1 1
  spline S856 degree 3 poles (50.4197, -69.1889) (50.6917, -68.8074) (50.8357, -68.3268) (50.8209, -67.8501) knots 0 0 0 0 1 1 1 1
  spline S857 degree 3 poles (50.8209, -67.8501) (50.8061, -67.3735) (50.6327, -66.9039) (50.3379, -66.5419) knots 0 0 0 0 1 1 1 1
  spline S858 degree 3 poles (50.3379, -66.5419) (50.043, -66.1798) (49.6286, -65.9278) (49.1833, -65.8396) knots 0 0 0 0 1 1 1 1
  line L251 (49.1833, -65.8396) -> (40.0515, -65.8778)
  spline S859 degree 3 poles (39.4762, -92.3793) (39.332, -92.3686) (39.1847, -92.4122) (39.0669, -92.5004) knots 0 0 0 0 1 1 1 1
  spline S860 degree 3 poles (39.0669, -92.5004) (38.9354, -92.5989) (38.8424, -92.7524) (38.8129, -92.9193) knots 0 0 0 0 1 1 1 1
  line L252 (38.8129, -92.9193) -> (38.7891, -95.6892)
  spline S861 degree 3 poles (38.7891, -95.6892) (38.7816, -95.8952) (38.8548, -96.1032) (38.9881, -96.2543) knots 0 0 0 0 1 1 1 1
  spline S862 degree 3 poles (38.9881, -96.2543) (39.1429, -96.4298) (39.3771, -96.524) (39.6037, -96.5019) knots 0 0 0 0 1 1 1 1
  line L253 (39.6037, -96.5019) -> (48.7355, -96.4703)
  spline S863 degree 3 poles (48.7355, -96.4703) (49.1745, -96.3519) (49.5725, -96.072) (49.8445, -95.6904) knots 0 0 0 0 1 1 1 1
  spline S864 degree 3 poles (49.8445, -95.6904) (50.1164, -95.3089) (50.2604, -94.8284) (50.2456, -94.3516) knots 0 0 0 0 1 1 1 1
  spline S865 degree 3 poles (50.2456, -94.3516) (50.2309, -93.875) (50.0575, -93.4054) (49.7626, -93.0434) knots 0 0 0 0 1 1 1 1
  spline S866 degree 3 poles (49.7626, -93.0434) (49.4677, -92.6813) (49.0533, -92.4293) (48.608, -92.3411) knots 0 0 0 0 1 1 1 1
  line L254 (48.608, -92.3411) -> (39.4762, -92.3793)
  spline S867 degree 3 poles (120.9407, -94.9113) (120.7967, -94.8988) (120.6488, -94.9405) (120.53, -95.0272) knots 0 0 0 0 1 1 1 1
  spline S868 degree 3 poles (120.53, -95.0272) (120.3975, -95.124) (120.3027, -95.2763) (120.2713, -95.4429) knots 0 0 0 0 1 1 1 1
  line L255 (120.2713, -95.4429) -> (120.2157, -98.2123)
  spline S869 degree 3 poles (120.2157, -98.2123) (120.2061, -98.4182) (120.2766, -98.6271) (120.4082, -98.7799) knots 0 0 0 0 1 1 1 1
  spline S870 degree 3 poles (120.4082, -98.7799) (120.561, -98.9573) (120.7941, -99.0545) (121.0209, -99.0353) knots 0 0 0 0 1 1 1 1
  line L256 (121.0209, -99.0353) -> (130.1525, -99.1196)
  spline S871 degree 3 poles (130.1525, -99.1196) (130.5927, -99.0068) (130.994, -98.732) (131.2703, -98.3539) knots 0 0 0 0 1 1 1 1
  spline S872 degree 3 poles (131.2703, -98.3539) (131.5465, -97.9758) (131.696, -97.4971) (131.6867, -97.0203) knots 0 0 0 0 1 1 1 1
  spline S873 degree 3 poles (131.6867, -97.0203) (131.6772, -96.5435) (131.5094, -96.0717) (131.2187, -95.706) knots 0 0 0 0 1 1 1 1
  spline S874 degree 3 poles (131.2187, -95.706) (130.928, -95.3402) (130.5165, -95.0829) (130.0723, -94.9891) knots 0 0 0 0 1 1 1 1
  line L257 (130.0723, -94.9891) -> (120.9407, -94.9113)
  spline S875 degree 3 poles (121.5841, -68.169) (121.4392, -68.1599) (121.2917, -68.2048) (121.1739, -68.2942) knots 0 0 0 0 1 1 1 1
  spline S876 degree 3 poles (121.1739, -68.2942) (121.0371, -68.3981) (120.9423, -68.5614) (120.917, -68.737) knots 0 0 0 0 1 1 1 1
  line L258 (120.917, -68.737) -> (120.8736, -71.6787)
  spline S877 degree 3 poles (120.8736, -71.6787) (120.8582, -71.8959) (120.9304, -72.1184) (121.0686, -72.2805) knots 0 0 0 0 1 1 1 1
  spline S878 degree 3 poles (121.0686, -72.2805) (121.2216, -72.4599) (121.4537, -72.5613) (121.6824, -72.5487) knots 0 0 0 0 1 1 1 1
  line L259 (121.6824, -72.5487) -> (130.8142, -72.5912)
  spline S879 degree 3 poles (130.8142, -72.5912) (131.2614, -72.4454) (131.6609, -72.1424) (131.9338, -71.742) knots 0 0 0 0 1 1 1 1
  spline S880 degree 3 poles (131.9338, -71.742) (132.2067, -71.3416) (132.3514, -70.8462) (132.3393, -70.3536) knots 0 0 0 0 1 1 1 1
  spline S881 degree 3 poles (132.3393, -70.3536) (132.3272, -69.8627) (132.1596, -69.3775) (131.8692, -68.9932) knots 0 0 0 0 1 1 1 1
  spline S882 degree 3 poles (131.8692, -68.9932) (131.5789, -68.6088) (131.1676, -68.3276) (130.716, -68.2046) knots 0 0 0 0 1 1 1 1
  line L260 (130.716, -68.2046) -> (121.5841, -68.169)
  spline S883 degree 3 poles (50.9385, -73.4216) (50.7451, -73.3668) (50.5295, -73.3948) (50.3608, -73.5083) knots 0 0 0 0 1 1 1 1
  spline S884 degree 3 poles (50.3608, -73.5083) (50.2764, -73.5651) (50.2043, -73.6422) (50.1531, -73.7327) knots 0 0 0 0 1 1 1 1
  spline S885 degree 3 poles (50.1531, -73.7327) (50.1018, -73.8233) (50.0718, -73.9272) (50.0679, -74.0325) knots 0 0 0 0 1 1 1 1
  spline S886 degree 3 poles (50.0679, -74.0325) (50.0641, -74.1357) (50.0855, -74.2395) (50.128, -74.3325) knots 0 0 0 0 1 1 1 1
  spline S887 degree 3 poles (50.128, -74.3325) (50.1706, -74.4255) (50.2342, -74.5075) (50.3113, -74.5713) knots 0 0 0 0 1 1 1 1
  spline S888 degree 3 poles (50.3113, -74.5713) (50.4655, -74.6989) (50.6719, -74.7499) (50.866, -74.7198) knots 0 0 0 0 1 1 1 1
  spline S889 degree 3 poles (50.866, -74.7198) (51.0123, -74.6972) (51.1533, -74.6293) (51.2598, -74.5212) knots 0 0 0 0 1 1 1 1
  spline S890 degree 3 poles (51.2598, -74.5212) (51.3663, -74.4131) (51.4366, -74.2643) (51.4464, -74.1089) knots 0 0 0 0 1 1 1 1
  spline S891 degree 3 poles (51.4464, -74.1089) (51.4562, -73.952) (51.404, -73.7933) (51.3102, -73.6709) knots 0 0 0 0 1 1 1 1
  spline S892 degree 3 poles (51.3102, -73.6709) (51.2164, -73.5486) (51.0828, -73.4624) (50.9385, -73.4216) knots 0 0 0 0 1 1 1 1
  spline S893 degree 3 poles (50.6842, -88.2085) (50.4908, -88.1537) (50.2752, -88.1817) (50.1065, -88.2952) knots 0 0 0 0 1 1 1 1
  spline S894 degree 3 poles (50.1065, -88.2952) (50.0221, -88.352) (49.95, -88.4291) (49.8987, -88.5196) knots 0 0 0 0 1 1 1 1
  spline S895 degree 3 poles (49.8987, -88.5196) (49.8475, -88.6102) (49.8174, -88.7141) (49.8136, -88.8194) knots 0 0 0 0 1 1 1 1
  spline S896 degree 3 poles (49.8136, -88.8194) (49.8097, -88.9226) (49.8311, -89.0264) (49.8737, -89.1194) knots 0 0 0 0 1 1 1 1
  spline S897 degree 3 poles (49.8737, -89.1194) (49.9163, -89.2124) (49.9799, -89.2944) (50.057, -89.3582) knots 0 0 0 0 1 1 1 1
  spline S898 degree 3 poles (50.057, -89.3582) (50.2112, -89.4858) (50.4176, -89.5368) (50.6116, -89.5068) knots 0 0 0 0 1 1 1 1
  spline S899 degree 3 poles (50.6116, -89.5068) (50.758, -89.4841) (50.899, -89.4162) (51.0055, -89.3081) knots 0 0 0 0 1 1 1 1
  spline S900 degree 3 poles (51.0055, -89.3081) (51.112, -89.2) (51.1823, -89.0512) (51.1921, -88.8958) knots 0 0 0 0 1 1 1 1
  spline S901 degree 3 poles (51.1921, -88.8958) (51.2019, -88.7389) (51.1497, -88.5802) (51.0559, -88.4578) knots 0 0 0 0 1 1 1 1
  spline S902 degree 3 poles (51.0559, -88.4578) (50.962, -88.3355) (50.8284, -88.2493) (50.6842, -88.2085) knots 0 0 0 0 1 1 1 1
  spline S903 degree 3 poles (120.117, -75.6839) (119.9237, -75.6291) (119.7081, -75.6572) (119.5393, -75.7706) knots 0 0 0 0 1 1 1 1
  spline S904 degree 3 poles (119.5393, -75.7706) (119.455, -75.8274) (119.3828, -75.9045) (119.3316, -75.9951) knots 0 0 0 0 1 1 1 1
  spline S905 degree 3 poles (119.3316, -75.9951) (119.2804, -76.0856) (119.2503, -76.1895) (119.2464, -76.2948) knots 0 0 0 0 1 1 1 1
  spline S906 degree 3 poles (119.2464, -76.2948) (119.2422, -76.398) (119.264, -76.5018) (119.3066, -76.5948) knots 0 0 0 0 1 1 1 1
  spline S907 degree 3 poles (119.3066, -76.5948) (119.3492, -76.6878) (119.4128, -76.7698) (119.4899, -76.8336) knots 0 0 0 0 1 1 1 1
  spline S908 degree 3 poles (119.4899, -76.8336) (119.644, -76.9612) (119.8505, -77.0122) (120.0445, -76.9822) knots 0 0 0 0 1 1 1 1
  spline S909 degree 3 poles (120.0445, -76.9822) (120.1909, -76.9595) (120.3319, -76.8916) (120.4384, -76.7835) knots 0 0 0 0 1 1 1 1
  spline S910 degree 3 poles (120.4384, -76.7835) (120.5449, -76.6754) (120.6152, -76.5266) (120.6249, -76.3712) knots 0 0 0 0 1 1 1 1
  spline S911 degree 3 poles (120.6249, -76.3712) (120.6345, -76.2143) (120.5825, -76.0556) (120.4887, -75.9333) knots 0 0 0 0 1 1 1 1
  spline S912 degree 3 poles (120.4887, -75.9333) (120.395, -75.8109) (120.2613, -75.7247) (120.117, -75.6839) knots 0 0 0 0 1 1 1 1
  spline S913 degree 3 poles (119.7543, -90.3468) (119.5609, -90.292) (119.3453, -90.3201) (119.1766, -90.4336) knots 0 0 0 0 1 1 1 1
  spline S914 degree 3 poles (119.1766, -90.4336) (119.0922, -90.4903) (119.02, -90.5674) (118.9688, -90.658) knots 0 0 0 0 1 1 1 1
  spline S915 degree 3 poles (118.9688, -90.658) (118.9177, -90.7485) (118.8876, -90.8525) (118.8836, -90.9578) knots 0 0 0 0 1 1 1 1
  spline S916 degree 3 poles (118.8836, -90.9578) (118.8794, -91.0609) (118.9012, -91.1648) (118.9438, -91.2577) knots 0 0 0 0 1 1 1 1
  spline S917 degree 3 poles (118.9438, -91.2577) (118.9864, -91.3507) (119.05, -91.4327) (119.1271, -91.4965) knots 0 0 0 0 1 1 1 1
  spline S918 degree 3 poles (119.1271, -91.4965) (119.2813, -91.6241) (119.4877, -91.6751) (119.6817, -91.6451) knots 0 0 0 0 1 1 1 1
  spline S919 degree 3 poles (119.6817, -91.6451) (119.8281, -91.6225) (119.9691, -91.5546) (120.0756, -91.4464) knots 0 0 0 0 1 1 1 1
  spline S920 degree 3 poles (120.0756, -91.4464) (120.1821, -91.3383) (120.2524, -91.1895) (120.2622, -91.0341) knots 0 0 0 0 1 1 1 1
  spline S921 degree 3 poles (120.2622, -91.0341) (120.2717, -90.8773) (120.2198, -90.7185) (120.126, -90.5962) knots 0 0 0 0 1 1 1 1
  spline S922 degree 3 poles (120.126, -90.5962) (120.0322, -90.4738) (119.8985, -90.3877) (119.7543, -90.3468) knots 0 0 0 0 1 1 1 1
  spline S923 degree 3 poles (49.0349, -107.9076) (49.891, -106.9233) (48.8117, -104.7507) (49.8436, -104.7415) knots 0 0 0 0 1 1 1 1
  spline S924 degree 3 poles (49.8436, -104.7415) (54.9196, -104.6966) (66.1899, -104.2774) (68.0171, -104.8389) knots 0 0 0 0 1 1 1 1
  spline S925 degree 3 poles (68.0171, -104.8389) (70.5962, -105.6315) (72.4242, -106.5648) (75.0106, -108.8816) knots 0 0 0 0 1 1 1 1
  spline S926 degree 3 poles (75.0106, -108.8816) (76.1744, -109.9242) (76.5239, -112.2771) (76.1048, -113.8011) knots 0 0 0 0 1 1 1 1
  spline S927 degree 3 poles (76.1048, -113.8011) (75.5497, -115.8193) (73.5493, -117.3585) (72.2037, -117.5029) knots 0 0 0 0 1 1 1 1
  spline S928 degree 3 poles (72.2037, -117.5029) (69.471, -117.7961) (63.864, -117.4546) (59.7391, -117.99) knots 0 0 0 0 1 1 1 1
  spline S929 degree 3 poles (59.7391, -117.99) (58.9985, -118.0861) (58.2896, -118.3681) (57.5507, -118.4771) knots 0 0 0 0 1 1 1 1
  spline S930 degree 3 poles (57.5507, -118.4771) (56.6851, -118.6049) (55.7711, -118.4123) (54.9341, -118.6717) knots 0 0 0 0 1 1 1 1
  spline S931 degree 3 poles (54.9341, -118.6717) (53.4863, -119.1203) (52.1039, -121.0992) (50.9854, -120.961) knots 0 0 0 0 1 1 1 1
  spline S932 degree 3 poles (50.9854, -120.961) (49.3598, -120.7601) (44.1147, -113.0104) (44.2773, -111.3168) knots 0 0 0 0 1 1 1 1
  spline S933 degree 3 poles (44.2773, -111.3168) (44.5587, -109.8625) (48.3225, -108.7265) (49.0349, -107.9076) knots 0 0 0 0 1 1 1 1
  spline S934 degree 3 poles (70.824, -108.7357) (69.2774, -108.8037) (67.5034, -110.2685) (67.6365, -112.1939) knots 0 0 0 0 1 1 1 1
  spline S935 degree 3 poles (67.6365, -112.1939) (67.7545, -113.9005) (69.3037, -115.9308) (71.2522, -115.7496) knots 0 0 0 0 1 1 1 1
  spline S936 degree 3 poles (71.2522, -115.7496) (73.1778, -115.5706) (74.4346, -113.8711) (74.3445, -111.9503) knots 0 0 0 0 1 1 1 1
  spline S937 degree 3 poles (74.3445, -111.9503) (74.2436, -109.8003) (72.3949, -108.6664) (70.824, -108.7357) knots 0 0 0 0 1 1 1 1
  spline S938 degree 3 poles (65.3203, -114.9374) (65.0267, -114.9456) (64.6899, -115.2157) (64.7152, -115.5654) knots 0 0 0 0 1 1 1 1
  spline S939 degree 3 poles (64.7152, -115.5654) (64.7378, -115.8752) (65.0317, -116.2441) (65.4016, -116.2112) knots 0 0 0 0 1 1 1 1
  spline S940 degree 3 poles (65.4016, -116.2112) (65.7671, -116.1782) (66.0057, -115.8701) (65.9886, -115.5212) knots 0 0 0 0 1 1 1 1
  spline S941 degree 3 poles (65.9886, -115.5212) (65.9697, -115.1307) (65.6185, -114.9248) (65.3203, -114.9374) knots 0 0 0 0 1 1 1 1
  spline S942 degree 3 poles (67.366, -105.9751) (67.0724, -105.9834) (66.7356, -106.2535) (66.7609, -106.6032) knots 0 0 0 0 1 1 1 1
  spline S943 degree 3 poles (66.7609, -106.6032) (66.7835, -106.9129) (67.0775, -107.2818) (67.4473, -107.2489) knots 0 0 0 0 1 1 1 1
  spline S944 degree 3 poles (67.4473, -107.2489) (67.8129, -107.216) (68.0514, -106.9079) (68.0343, -106.559) knots 0 0 0 0 1 1 1 1
  spline S945 degree 3 poles (68.0343, -106.559) (68.0154, -106.1685) (67.6643, -105.9626) (67.366, -105.9751) knots 0 0 0 0 1 1 1 1
  line L261 (48.7256, -112.5592) -> (51.0806, -111.2441)
  line L262 (51.0806, -111.2441) -> (53.3403, -114.7997)
  line L263 (53.3403, -114.7997) -> (50.9378, -116.3584)
  line L264 (50.9378, -116.3584) -> (48.7256, -112.5592)
  spline S946 degree 3 poles (16.5948, -70.3631) (17.0596, -70.4153) (18.3456, -72.3953) (18.7586, -72.399) knots 0 0 0 0 1 1 1 1
  spline S947 degree 3 poles (18.7586, -72.399) (19.1152, -72.4023) (19.2557, -72.0363) (19.4963, -72.0766) knots 0 0 0 0 1 1 1 1
  spline S948 degree 2 poles (19.4963, -72.0766) (21.0931, -73.9205) (20.5922, -74.6731) knots 0 0 0 1 1 1
  spline S949 degree 3 poles (20.5922, -74.6731) (11.5856, -88.2037) (13.0359, -100.4596) (14.1139, -117.6298) knots 0 0 0 0 1 1 1 1
  spline S950 degree 3 poles (14.1139, -117.6298) (14.3258, -121.0056) (14.2396, -124.4784) (13.6887, -127.8297) knots 0 0 0 0 1 1 1 1
  spline S951 degree 3 poles (13.6887, -127.8297) (11.3921, -141.7999) (8.6828, -152.0581) (17.3817, -168.3098) knots 0 0 0 0 1 1 1 1
  spline S952 degree 3 poles (17.3817, -168.3098) (17.6796, -168.8665) (16.4006, -169.7037) (16.0365, -169.8495) knots 0 0 0 0 1 1 1 1
  spline S953 degree 3 poles (16.0365, -169.8495) (15.6731, -169.9946) (15.1423, -169.618) (14.7424, -169.8128) knots 0 0 0 0 1 1 1 1
  spline S954 degree 3 poles (14.7424, -169.8128) (14.3696, -169.9962) (13.7486, -171.1384) (13.2952, -171.2557) knots 0 0 0 0 1 1 1 1
  spline S955 degree 3 poles (13.2952, -171.2557) (12.8583, -171.3686) (10.879, -169.3642) (10.8886, -168.9415) knots 0 0 0 0 1 1 1 1
  spline S956 degree 3 poles (10.8886, -168.9415) (10.896, -168.6163) (11.7786, -167.5089) (11.9887, -166.6517) knots 0 0 0 0 1 1 1 1
  spline S957 degree 3 poles (11.9887, -166.6517) (11.2706, -165.7993) (11.2126, -165.7625) (10.7075, -165.2382) knots 0 0 0 0 1 1 1 1
  spline S958 degree 3 poles (10.7075, -165.2382) (9.5266, -165.6039) (9.0816, -166.5872) (8.5071, -166.5593) knots 0 0 0 0 1 1 1 1
  spline S959 degree 3 poles (8.5071, -166.5593) (7.973, -166.5349) (6.9985, -165.8194) (6.9024, -165.4664) knots 0 0 0 0 1 1 1 1
  spline S960 degree 3 poles (6.9024, -165.4664) (3.7467, -145.2562) (8.8562, -139.3012) (9.7611, -126.2073) knots 0 0 0 0 1 1 1 1
  spline S961 degree 3 poles (9.7611, -126.2073) (10.6602, -113.198) (8.9788, -109.1726) (8.2823, -97.2392) knots 0 0 0 0 1 1 1 1
  spline S962 degree 3 poles (8.2823, -97.2392) (7.8969, -90.6379) (7.0048, -89.8791) (10.8016, -74.8638) knots 0 0 0 0 1 1 1 1
  spline S963 degree 3 poles (10.8016, -74.8638) (11.3432, -74.3206) (12.6572, -76.3498) (13.5809, -76.8592) knots 0 0 0 0 1 1 1 1
  spline S964 degree 3 poles (13.5809, -76.8592) (14.8954, -76.0668) (14.903, -76.024) (15.8017, -75.1575) knots 0 0 0 0 1 1 1 1
  spline S965 degree 3 poles (15.8017, -75.1575) (15.1075, -74.2259) (14.3369, -72.9845) (14.3128, -72.636) knots 0 0 0 0 1 1 1 1
  spline S966 degree 3 poles (14.3128, -72.636) (14.2871, -72.2659) (16.1831, -70.315) (16.5948, -70.3614) knots 0 0 0 0 1 1 1 1
  line L265 (16.5948, -70.3614) -> (16.5948, -70.3631)
  spline S967 degree 3 poles (82.8462, -15.7383) (83.237, -15.149) (83.7364, -14.632) (84.3118, -14.221) knots 0 0 0 0 1 1 1 1
  spline S968 degree 3 poles (84.3118, -14.221) (85.5163, -13.3607) (87.0031, -12.9917) (88.4707, -12.7988) knots 0 0 0 0 1 1 1 1
  spline S969 degree 3 poles (88.4707, -12.7988) (90.9014, -12.4793) (93.3862, -12.5966) (95.7825, -13.1147) knots 0 0 0 0 1 1 1 1
  spline S970 degree 3 poles (95.7825, -13.1147) (99.235, -13.861) (102.5001, -15.4433) (105.2454, -17.6659) knots 0 0 0 0 1 1 1 1
  spline S971 degree 3 poles (105.2454, -17.6659) (107.3923, -19.4042) (109.2239, -21.5308) (110.6245, -23.9117) knots 0 0 0 0 1 1 1 1
  line L266 (110.6245, -23.9117) -> (110.5681, -35.0892)
  line L267 (110.5681, -35.0892) -> (113.2963, -35.134)
  line L268 (113.2963, -35.134) -> (113.2283, -38.0774)
  line L269 (113.2283, -38.0774) -> (110.3523, -38.201)
  line L270 (110.3523, -38.201) -> (110.1673, -49.4365)
  spline S972 degree 3 poles (110.1673, -49.4365) (108.9539, -51.2185) (107.5146, -52.8464) (105.8947, -54.269) knots 0 0 0 0 1 1 1 1
  spline S973 degree 3 poles (105.8947, -54.269) (103.778, -56.1279) (101.3269, -57.6457) (98.63, -58.4599) knots 0 0 0 0 1 1 1 1
  spline S974 degree 3 poles (98.63, -58.4599) (96.6572, -59.0555) (94.5889, -59.267) (92.5306, -59.3664) knots 0 0 0 0 1 1 1 1
  spline S975 degree 3 poles (92.5306, -59.3664) (89.816, -59.4976) (86.9692, -59.4088) (84.5792, -58.1148) knots 0 0 0 0 1 1 1 1
  spline S976 degree 3 poles (84.5792, -58.1148) (83.4971, -57.529) (82.5434, -56.7075) (81.8039, -55.7241) knots 0 0 0 0 1 1 1 1
  line L271 (81.8039, -55.7241) -> (92.3921, -55.7608)
  line L272 (92.3921, -55.7608) -> (93.0494, -43.1969)
  line L273 (93.0494, -43.1969) -> (97.5569, -43.1076)
  line L274 (97.5569, -43.1076) -> (97.8622, -29.0004)
  line L275 (97.8622, -29.0004) -> (93.1622, -28.9205)
  line L276 (93.1622, -28.9205) -> (92.9697, -15.7253)
  line L277 (92.9697, -15.7253) -> (82.8462, -15.7383)
  spline S977 degree 3 poles (23.587, -128.5774) (22.3853, -128.9147) (21.1124, -128.9713) (19.8877, -128.742) knots 0 0 0 0 1 1 1 1
  spline S978 degree 3 poles (19.8877, -128.742) (19.4755, -128.6648) (19.0665, -128.5548) (18.685, -128.374) knots 0 0 0 0 1 1 1 1
  spline S979 degree 3 poles (18.685, -128.374) (18.3035, -128.1933) (17.9492, -127.9392) (17.6806, -127.6033) knots 0 0 0 0 1 1 1 1
  spline S980 degree 3 poles (17.6806, -127.6033) (17.3144, -127.1455) (17.1241, -126.5587) (17.0298, -125.9701) knots 0 0 0 0 1 1 1 1
  spline S981 degree 3 poles (17.0298, -125.9701) (16.9354, -125.3815) (16.9297, -124.7819) (16.8891, -124.1866) knots 0 0 0 0 1 1 1 1
  spline S982 degree 3 poles (16.8891, -124.1866) (16.8507, -123.6216) (16.7807, -123.0575) (16.7915, -122.4912) knots 0 0 0 0 1 1 1 1
  spline S983 degree 3 poles (16.7915, -122.4912) (16.8023, -121.9249) (16.8989, -121.3476) (17.1709, -120.8578) knots 0 0 0 0 1 1 1 1
  spline S984 degree 3 poles (17.1709, -120.8578) (17.3734, -120.4931) (17.6704, -120.1865) (18.0216, -119.9795) knots 0 0 0 0 1 1 1 1
  spline S985 degree 3 poles (18.0216, -119.9795) (18.3728, -119.7724) (18.7774, -119.6654) (19.1805, -119.673) knots 0 0 0 0 1 1 1 1
  line L278 (19.1805, -119.673) -> (26.6926, -119.4144)
  spline S986 degree 3 poles (26.6926, -119.4144) (26.9897, -119.4044) (27.2876, -119.3954) (27.5816, -119.3501) knots 0 0 0 0 1 1 1 1
  spline S987 degree 3 poles (27.5816, -119.3501) (27.8756, -119.3048) (28.1684, -119.2204) (28.4219, -119.0581) knots 0 0 0 0 1 1 1 1
  spline S988 degree 3 poles (28.4219, -119.0581) (28.7716, -118.8344) (29.0316, -118.4622) (29.1292, -118.0459) knots 0 0 0 0 1 1 1 1
  line L279 (29.1292, -118.0459) -> (29.3784, -115.7746)
  spline S989 degree 3 poles (29.3784, -115.7746) (30.8177, -115.5227) (32.3103, -115.6094) (33.7142, -116.0265) knots 0 0 0 0 1 1 1 1
  spline S990 degree 3 poles (33.7142, -116.0265) (35.7865, -116.6422) (37.6755, -118.013) (38.8151, -119.925) knots 0 0 0 0 1 1 1 1
  spline S991 degree 3 poles (38.8151, -119.925) (39.5748, -121.1996) (39.9923, -122.6947) (40.0079, -124.1965) knots 0 0 0 0 1 1 1 1
  line L280 (40.0079, -124.1965) -> (40.4433, -131.2609)
  spline S992 degree 3 poles (40.4433, -131.2609) (40.5906, -131.9423) (40.9825, -132.5627) (41.524, -132.9717) knots 0 0 0 0 1 1 1 1
  spline S993 degree 3 poles (41.524, -132.9717) (41.8102, -133.188) (42.1374, -133.3443) (42.4809, -133.4301) knots 0 0 0 0 1 1 1 1
  spline S994 degree 3 poles (42.4809, -133.4301) (42.8244, -133.5158) (43.1803, -133.5265) (43.5334, -133.528) knots 0 0 0 0 1 1 1 1
  line L281 (43.5334, -133.528) -> (57.892, -133.59)
  spline S995 degree 3 poles (57.892, -133.59) (58.8549, -133.56) (59.8184, -134.0631) (60.3742, -134.8859) knots 0 0 0 0 1 1 1 1